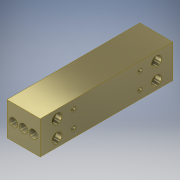
# Autodesk Inventor part: BottomOfBackElevatorFrame
Saved by Autodesk Inventor 2019 (Build 230136000, 136)
## iProperties
Created: 2019-09-28
Part Number: BottomOfBackElevatorFrame
Material: Generic
Document SubType Name: Modeling
Designer: james
Density: 1 g/cm^3
Appearance: Gold - Metal
Mass: 54.1046 g
Surface Area: 195.592 cm^2
Volume: 54.1046 cm^3
Author: james
Autodesk Inventor part; units mm, degrees
ref_plane "YZ Plane" through (0, 0, 0) normal (1, 0, 0) x (0, 1, 0)
ref_plane "XZ Plane" through (0, 0, 0) normal (0, 1, 0) x (-1, 0, 0)
ref_plane "XY Plane" through (0, 0, 0) normal (0, 0, 1) x (1, 0, 0)
sketch "Sketch1" plane through (0, 0, 0) normal (0, 0, 1) x (1, 0, 0)
  line L0 (-13.202, 13.202) -> (12.198, 13.202)
  line L1 (12.198, 13.202) -> (12.198, -12.198)
  line L2 (12.198, -12.198) -> (-13.202, -12.198)
  line L3 (-13.202, -12.198) -> (-13.202, 13.202)
  point P0 (0, 0)
  dimension "d0" = 25.4
  dimension "d1" = 25.4
  constraints: 8 end point, 2 parallel, 1 horizontal, 1 perpendicular
  measures "d0" distance of L1.end L2.end
  measures "d1" distance of L2.end L0.start
extrude "Extrusion1" add sketch "Sketch1" along normal blind 101.6
sketch "Sketch6" plane through (12.198, 13.202, 101.6) normal (1, 0, 0) x (0, 0, -1)
  line L0 (101.6, 0) -> (101.6, -25.4) projected
  line L1 (101.6, -25.4) -> (0, -25.4) projected
  line L2 (101.6, 0) -> (101.6, -25.4) projected
  line L3 (101.6, 0) -> (0, 0) projected
  line L4 (0, -25.4) -> (0, 0) projected
  line L5 (0, -25.4) -> (0, 0) projected
  point P0 (101.6, -13.202)
  point P1 (88.9, -6.35)
  point P2 (88.9, -19.05)
  point P3 (101.6, -19.05)
  point P4 (101.6, -6.35)
  point P5 (12.7, -6.35)
  point P6 (12.7, -19.05)
  point P7 (0, -19.05)
  point P8 (0, -6.35)
  dimension "d51" = 12.7
  dimension "d52" = 6.35
  dimension "d53" = 12.7
  dimension "d54" = 6.35
  dimension "d55" = 12.7
  dimension "d56" = 6.35
  dimension "d57" = 12.7
  dimension "d58" = 6.35
  measures "d51" distance from line of point (88.9, -19.05) L0
  measures "d52" distance from line of L1 point (88.9, -19.05)
  measures "d53" distance from line of L2 point (88.9, -6.35)
  measures "d54" distance from line of L3 point (88.9, -6.35)
  measures "d55" distance from line of L4 point (12.7, -19.05)
  measures "d56" distance from line of L1 point (12.7, -19.05)
  measures "d57" distance from line of L5 point (12.7, -6.35)
  measures "d58" distance from line of L3 point (12.7, -6.35)
sketch "Sketch7" plane through (12.198, 13.202, 101.6) normal (1, 0, 0) x (0, 0, -1)
  line L0 (0, -25.4) -> (0, 0) projected
  line L1 (101.6, 0) -> (0, 0) projected
  point P0 (101.6, -13.202)
  point P1 (25.4, -6.35)
  point P2 (25.4, -19.05)
  point P3 (76.2, -6.35)
  point P4 (76.2, -19.05)
  point P5 (0, -6.35)
  dimension "d66" = 0
  dimension "d67" = 0
  dimension "d68" = 0
  dimension "d69" = 0
  dimension "d70" = 25.4
  dimension "d71" = 6.35
  dimension "d72" = 19.05
  dimension "d73" = 76.2
  measures "d66" vertical distance of point (25.4, -19.05) point (76.2, -19.05)
  measures "d67" vertical distance of point (25.4, -6.35) point (76.2, -6.35)
  measures "d68" horizontal distance of point (76.2, -19.05) point (76.2, -6.35)
  measures "d69" horizontal distance of point (25.4, -6.35) point (25.4, -19.05)
  measures "d70" distance from line of point (25.4, -6.35) L0
  measures "d71" distance from line of L1 point (25.4, -6.35)
  measures "d72" distance from line of L1 point (25.4, -19.05)
  measures "d73" distance from line of point (76.2, -6.35) L0
hole "Hole3" at (12.198, 6.852, 76.2) at (12.198, -5.848, 76.2) at (12.198, 6.852, 25.4) at (12.198, -5.848, 25.4) direction (-1, 0, 0) diameter 3.175 depth 25.4 tip angle 118.188
sketch "Sketch8" plane through (0, 0, 101.6) normal (0, 0, 1) x (1, 0, 0)
  line L0 (-13.202, 13.202) -> (-13.202, -12.198) projected
  line L1 (-13.202, -12.198) -> (12.198, -12.198) projected
  point P0 (0, 0)
  point P1 (-8.122, 0.502)
  point P2 (-0.502, 0.502)
  point P3 (7.118, 0.502)
  dimension "d81" = 0
  dimension "d82" = 5.08
  dimension "d83" = 12.7
  dimension "d84" = 12.7
  dimension "d85" = 0
  dimension "d86" = 20.32
  measures "d81" vertical distance of point (-8.122, 0.502) point (-0.502, 0.502)
  measures "d82" distance from line of L0 point (-8.122, 0.502)
  measures "d83" distance from line of point (-0.502, 0.502) L0
  measures "d84" distance from line of L1 point (-8.122, 0.502)
  measures "d85" vertical distance of point (7.118, 0.502) point (-0.502, 0.502)
  measures "d86" distance from line of L0 point (7.118, 0.502)
hole "Hole4" at (-8.122, 0.502, 101.6) at (-0.502, 0.502, 101.6) at (7.118, 0.502, 101.6) direction (0, 0, -1) diameter 6.477 end through all
hole "Hole5" at (12.198, 6.852, 12.7) at (12.198, -5.848, 12.7) at (12.198, 6.852, 88.9) at (12.198, -5.848, 88.9) direction (-1, 0, 0) diameter 4.318 end through all counterbore diameter 7.62 counterbore depth 4.318
body "Solid1"
